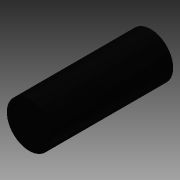
# Autodesk Inventor part: Gearbox Pin
Saved by Autodesk Inventor 2014 SP1 (Build 180222100, 222)
## iProperties
Created: 2013-05-05
Part Number: Gearbox Pin
Material: Steel
Document SubType Name: Modeling
Designer: Moses
Mass: 0.181232 g
Surface Area: 0.494174 cm^2
Volume: 0.0230868 cm^3
Density: 7.85 g/cm^3
Appearance: Anodized - Black
Author: Moses
Autodesk Inventor part; units mm, degrees
ref_plane "YZ Plane" through (0, 0, 0) normal (1, 0, 0) x (0, 1, 0)
ref_plane "XZ Plane" through (0, 0, 0) normal (0, 1, 0) x (-1, 0, 0)
ref_plane "XY Plane" through (0, 0, 0) normal (0, 0, 1) x (1, 0, 0)
sketch "Sketch1" plane through (0, 0, 0) normal (0, 0, 1) x (1, 0, 0)
  circle A0 centre (0, 0) radius 1.1067
  dimension "d0" = 2.2134
  constraints: 1 centre point, 1 coincident
  measures "d0" diameter of A0
extrude "Extrusion1" add sketch "Sketch1" along normal blind 6
body "Solid1"
